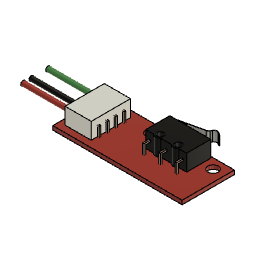
Endstop switch (Autodesk Fusion 360 design; units mm, degrees)
Autodesk Fusion 360 part; units mm, degrees
sketch "PCB" plane through (0, 0, 0) normal (0, 0, 1) x (1, 0, 0)
  line L0 (19.75, 8) -> (-19.75, 8)
  line L1 (-19.75, 8) -> (-19.75, -8)
  line L2 (-19.75, -8) -> (19.75, -8)
  line L3 (19.75, -8) -> (19.75, 8)
  line L4 (19.75, 8) -> (-19.75, -8) construction
  line L5 (-19.75, 8) -> (19.75, -8) construction
  line L6 (-6, 5) -> (19.75, 5) construction
  circle A0 centre (16.25, 5) radius 1.6
  circle A1 centre (-2.75, 5) radius 1.6
  dimension "d1" = 39.5
  dimension "d2" = 16
  dimension "d3" = 3
  dimension "d4" = 3.2
  dimension "d5" = 3.2
  dimension "d6" = 3.5
  dimension "d7" = 19
  constraint perpendicular L0 L1
  constraint parallel L0 L2
  constraint parallel L1 L3
  constraint horizontal L0
  constraint coincident L4 origin
  constraint coincident L5 origin
  constraint coincident L3 L6.end
  constraint perpendicular L3 L6
  constraint coincident L6 A0.centre
  constraint coincident L6 A1.centre
  measures "d1" distance of L1.end L2.end
  measures "d2" distance of L0.end L1.end
  measures "d3" distance of L0 L6
  measures "d4" diameter of A0
  measures "d5" diameter of A1
  measures "d6" distance of L3 A0.centre
  measures "d7" distance of A0.centre A1.centre
extrude "Extrude1" add sketch "PCB" along normal blind 1.2 makes body 1
sketch "Components" plane through (0, 0, 1.2) normal (0, 0, 1) x (-1, 0, 0)
  circle A0 centre (-16.25, -5) radius 1.6
  circle A1 centre (2.75, -5) radius 1.6
  line L0 (-19.75, 8) -> (-19.75, -8)
  line L1 (-19.75, -8) -> (19.75, -8)
  line L2 (19.75, -8) -> (19.75, 8)
  line L3 (19.75, 8) -> (-19.75, 8)
  line L4 (10, 6) -> (18, 6)
  line L5 (18, 6) -> (18, -6)
  line L6 (18, -6) -> (10, -6)
  line L7 (10, -6) -> (10, 6)
  line L8 (-0.5, -7.5) -> (-13, -7.5)
  line L9 (-13, -7.5) -> (-13, -0.1389)
  line L10 (-0.5, -0.1389) -> (-0.5, -7.5)
  circle A2 centre (-4, -1.1389) radius 1
  circle A3 centre (-9.5, -1.1389) radius 1
  line L11 (-2.882, -0.1389) -> (-0.5, -0.1389)
  line L12 (-13, -0.1389) -> (-10.618, -0.1389)
  line L13 (-8.382, -0.1389) -> (-5.118, -0.1389)
  arc A4 (-8.382, -0.1389) -> (-10.618, -0.1389) centre (-9.5, -1.1389) ccw
  arc A5 (-2.882, -0.1389) -> (-5.118, -0.1389) centre (-4, -1.1389) ccw
  line L14 (-4.25, -6) -> (-4.25, -12) construction
  circle A6 centre (-4.25, -8.25) radius 0.5
  line L15 (-4.75, -8.25) -> (-4.75, -7.5)
  line L16 (-3.75, -8.25) -> (-3.75, -7.5)
  line L17 (-1.8367, -8.4749) -> (-9.0467, -10.1221)
  line L18 (-10.0575, -10.353) -> (-10.0353, -10.4505)
  line L19 (-8.9808, -10.2096) -> (-1.8145, -8.5724)
  line L20 (-1.8145, -8.5724) -> (-1.8367, -8.4749)
  arc A7 (-1.8145, -8.5724) -> (-0.9595, -7.5) centre (-2.0595, -7.5) ccw
  arc A8 (-1.8367, -8.4749) -> (-1.0595, -7.5) centre (-2.0595, -7.5) ccw
  line L21 (-9.634, -10.7021) -> (-9.9002, -11.1854)
  line L22 (-10.3826, -12.0613) -> (-10.4702, -12.0131)
  line L23 (-9.9395, -11.0495) -> (-9.6999, -10.6146)
  line L24 (-9.5053, -10.2612) -> (-9.4177, -10.3095)
  line L25 (-11.2585, -11.5789) -> (-12.1345, -11.0964)
  line L26 (-12.1345, -11.0964) -> (-12.0862, -11.0088)
  line L27 (-12.0862, -11.0088) -> (-11.2979, -11.443)
  line L28 (-10.3344, -11.9737) -> (-10.3826, -12.0613)
  arc A9 (-8.9808, -10.2096) -> (-9.634, -10.7021) centre (-8.758, -11.1845) ccw
  arc A10 (-9.0467, -10.1221) -> (-9.6999, -10.6146) centre (-8.824, -11.097) ccw
  arc A11 (-11.2979, -11.443) -> (-9.9395, -11.0495) centre (-10.8155, -10.5671) ccw
  arc A12 (-11.2585, -11.5789) -> (-9.9002, -11.1854) centre (-10.7761, -10.7029) ccw
  dimension "d10" = 15.5
  dimension "d11" = 1
  dimension "d12" = 0.75
  dimension "d13" = 0.5
  dimension "d21" = 2
  dimension "d22" = 2.2
  dimension "d33" = 2
  dimension "d34" = 0.1
  dimension "d35" = 0.1
  dimension "d36" = 1
  dimension "d37" = 1
  dimension "d38" = 1
  dimension "d39" = 1
  constraint horizontal L4
  constraint vertical L5
  constraint horizontal L6
  constraint vertical L7
  constraint horizontal L8
  constraint vertical L9
  constraint horizontal L12
  constraint vertical L10
  constraint tangent A2 L12
  constraint tangent A3 L12
  constraint concentric A2 A5
  constraint concentric A3 A4
  constraint collinear L11 L12
  constraint collinear L12 L13
  constraint perpendicular L1 L14
  constraint coincident L14 A6.centre
  constraint coincident A6 L15.start
  constraint coincident L8 L15.end
  constraint tangent A6 L15
  constraint perpendicular L8 L15
  constraint coincident A6 L16.start
  constraint coincident L8 L16.end
  constraint tangent A6 L16
  constraint perpendicular L8 L16
  constraint coincident L8 A7.centre
  constraint concentric A7 A8
  constraint perpendicular L17 L18
  constraint parallel L17 L19
  constraint parallel L18 L20
  constraint tangent L19 A7
  constraint tangent L17 A8
  constraint coincident L8 A8.end
  constraint coincident L8 A7.end
  constraint perpendicular L21 L22
  constraint parallel L21 L23
  constraint parallel L22 L24
  constraint coincident L19 L24.end
  constraint perpendicular L25 L26
  constraint parallel L25 L27
  constraint parallel L26 L28
  constraint perpendicular L23 L25
  constraint coincident L18.end L19
  constraint coincident L24.end L21
  constraint tangent L19 A9
  constraint tangent L21 A9
  constraint coincident L18.start L17
  constraint coincident L24.start L23
  constraint tangent L17 A10
  constraint tangent L23 A10
  constraint coincident L22.end L23
  constraint coincident L28.start L27
  constraint tangent L23 A11
  constraint tangent L27 A11
  constraint coincident L22.start L21
  constraint coincident L22.start L25
  constraint tangent L21 A12
  constraint tangent L25 A12
  measures "d10" distance of L0 L14
  measures "d11" diameter of A6
  measures "d12" distance of L8 A6.centre
  measures "d13" distance of L1 L8
  measures "d21" diameter of A8
  measures "d22" diameter of A7
  measures "d33" distance of L24.end L22.start
  measures "d34" distance of L24.end L24.start
  measures "d35" distance of L22.start L28.start
  measures "d36" radius of A9
  measures "d37" radius of A10
  measures "d38" radius of A11
  measures "d39" radius of A12
extrude "Extrude2" add sketch "Components" along normal blind 5 separate body contours L4 L5 L6 L7 makes body 2
extrude "Extrude3" add sketch "Components" along normal blind 5 separate body contours L8 L9 L10 L11 L12 L13 A4 A5 makes body 3
extrude "Extrude4" add sketch "Components" along normal blind 3 from surface at 1 separate body contours L1 L8 A6 L15 L16 | L1 A6 L15 | L1 A6 | L1 A6 | L1 A6 L16 makes body 4
extrude "Extrude5" add sketch "Components" along normal blind 3 from surface at 1 separate body contours L1 L20 A7 A8 | L1 L8 A7 A8 | L17 L19 L20 L21 L23 L25 L26 L27 A9 A10 A11 A12 makes body 5
sketch "Sketch3" plane through (-18, 0, 0) normal (-1, 0, 0) x (0, -1, 0)
  line L0 (-6, 1.2) -> (6, 1.2)
  line L1 (6, 1.2) -> (6, 6.2)
  line L2 (6, 6.2) -> (-6, 6.2)
  line L3 (-6, 6.2) -> (-6, 1.2)
  line L4 (-6, 3.7) -> (6, 3.7) construction
  circle A0 centre (1.27, 3.7) radius 0.75
  circle A1 centre (-3.81, 3.7) radius 0.75
  circle A2 centre (3.81, 3.7) radius 0.75
  dimension "d26" = 1.5
  dimension "d27" = 1.5
  dimension "d28" = 1.5
  dimension "d29" = 5.08
  dimension "d30" = 2.54
  constraint midpoint L3 L4.start
  constraint midpoint L1 L4.end
  constraint coincident L4 A1.centre
  constraint coincident L4 A2.centre
  measures "d26" diameter of A0
  measures "d27" diameter of A1
  measures "d28" diameter of A2
  measures "d29" distance of A0.centre A1.centre
  measures "d30" distance of A0.centre A2.centre
extrude "Extrude6" add sketch "Sketch3" along normal blind 15 contours A0 | A1 | A2 bodies 2
sketch "Switch legs" plane through (13, 0, 0) normal (1, 0, 0) x (0, 1, 0)
  line L0 (0.1389, 1.2) -> (7.5, 1.2)
  line L1 (7.5, 1.2) -> (7.5, 6.2)
  line L2 (7.5, 6.2) -> (0.1389, 6.2)
  line L3 (0.1389, 6.2) -> (0.1389, 1.2)
  line L4 (0.1389, 3.7) -> (-1.3611, 3.7)
  line L5 (-1.8611, 3.7) -> (-1.8611, 4.2)
  line L6 (-1.8611, 4.2) -> (0.1389, 4.2)
  line L7 (0.1389, 4.2) -> (0.1389, 3.7)
  line L8 (-1.8611, 4.2) -> (-1.3611, 4.2)
  line L9 (-1.3611, 3.7) -> (-1.3611, -1.8)
  line L10 (-1.3611, -1.8) -> (-1.8611, -1.8)
  line L11 (-1.8611, -1.8) -> (-1.8611, 4.2)
  dimension "d40" = 2
  dimension "d41" = 0.5
  dimension "d42" = 6
  dimension "d43" = 0.5
  constraint horizontal L4
  constraint vertical L5
  constraint horizontal L6
  constraint vertical L7
  constraint midpoint L3 L4.start
  constraint horizontal L8
  constraint vertical L9
  constraint horizontal L10
  constraint vertical L11
  measures "d40" distance of L4.start L5.start
  measures "d41" distance of L4.start L6.end
  measures "d42" distance of L5.end L10.end
  measures "d43" distance of L5.end L8.end
extrude "Extrude7" add sketch "Switch legs" against normal blind 0.5 from surface at -1 separate body contours L3 L4 L5 L6 L7 L8 L9 L10 L11 makes body 6
extrude "Extrude8" add sketch "Switch legs" against normal blind 0.5 from surface at -6 separate body contours L3 L4 L5 L6 L7 L8 L9 L10 L11 makes body 7
extrude "Extrude9" add sketch "Switch legs" against normal blind 0.5 from surface at -11 separate body contours L3 L4 L5 L6 L7 L8 L9 L10 L11 makes body 8
copy_body "CopyPasteBodies1" bodies 6 makes body 9
move_body "Move1" bodies 9 to x (0, 1, 0) y (-1, 0, 0) z (0, 0, 1) at (-11.3611, -15.5648, 0)
copy_body "CopyPasteBodies2" bodies 9 makes body 10
move_body "Move2" bodies 10 to x (1, 0, 0) y (0, 1, 0) z (0, 0, 1) at (0, 2.54, 0)
copy_body "CopyPasteBodies3" bodies 10 makes body 11
move_body "Move3" bodies 11 to x (1, 0, 0) y (0, 1, 0) z (0, 0, 1) at (0, 2.54, 0)
copy_body "CopyPasteBodies4" bodies 11 makes body 12
move_body "Move4" bodies 12 to x (1, 0, 0) y (0, 1, 0) z (0, 0, 1) at (0, 2.54, 0)
named bodies: "PCB", "Connector", "Switch body", "Switch", "Lever", "Switch leg 1", "Switch leg 2", "Switch leg 3", "Plug leg 1", "Plug leg 2", "Plug leg 3", "Plug leg 3 (1)"
